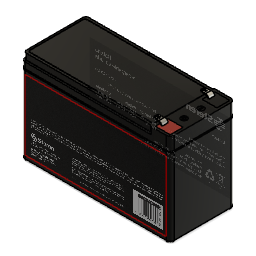
Batery-BR-1207-Steren v4 (Autodesk Fusion 360 design; units mm, degrees)
Autodesk Fusion 360 part; units mm, degrees
sketch "Sketch1" plane through (0, 0, 0) normal (0, 1, 0) x (1, 0, 0)
  line L0 (71, -32.5) -> (-71, -32.5)
  line L1 (-75, -28.5) -> (-75, 28.5)
  line L2 (-71, 32.5) -> (71, 32.5)
  line L3 (75, 28.5) -> (75, -28.5)
  line L4 (75, -32.5) -> (-75, 32.5) construction
  line L5 (-75, -32.5) -> (75, 32.5) construction
  arc A0 (-71, 32.5) -> (-75, 28.5) centre (-71, 28.5) ccw
  arc A1 (75, 28.5) -> (71, 32.5) centre (71, 28.5) ccw
  arc A2 (71, -32.5) -> (75, -28.5) centre (71, -28.5) ccw
  arc A3 (-75, -28.5) -> (-71, -32.5) centre (-71, -28.5) ccw
  dimension "d1" = 150
  dimension "d2" = 65
  dimension "d3" = 4
  constraint horizontal L0
  constraint perpendicular L0 L1
  constraint parallel L0 L2
  constraint parallel L1 L3
  constraint coincident L4 origin
  constraint coincident L5 origin
  constraint coincident L4.end L2
  constraint coincident L4.end L1
  constraint tangent L2 A0
  constraint tangent L1 A0
  constraint coincident L5.end L2
  constraint coincident L5.end L3
  constraint tangent L2 A1
  constraint tangent L3 A1
  constraint equal A0 A1
  constraint coincident L4.start L3
  constraint coincident L4.start L0
  constraint tangent L3 A2
  constraint tangent L0 A2
  constraint equal A0 A2
  constraint coincident L5.start L0
  constraint coincident L5.start L1
  constraint tangent L0 A3
  constraint tangent L1 A3
  constraint equal A0 A3
  measures "d1" distance of L4.end L5.end
  measures "d2" distance of L5.start L4.end
  measures "d3" radius of A0
extrude "Extrude1" add sketch "Sketch1" along normal blind 79 makes body 1
fillet "Fillet1" radius 2 8 edges at (75, 0, 0) (73.8284, 0, -31.3284) (0, 0, -32.5) (-73.8284, 0, -31.3284) (-75, 0, 0) (-73.8284, 0, 31.3284) (0, 0, 32.5) (73.8284, 0, 31.3284) on bodies 1
sketch "Sketch2" plane through (0, 0, 0) normal (0, -1, 0) x (1, 0, 0)
  line L0 (73, -28.5) -> (73, 28.5)
  arc A0 (73, 28.5) -> (71, 30.5) centre (71, 28.5) ccw
  line L1 (71, 30.5) -> (-71, 30.5)
  arc A1 (-71, 30.5) -> (-73, 28.5) centre (-71, 28.5) ccw
  line L2 (-73, 28.5) -> (-73, -28.5)
  arc A2 (-73, -28.5) -> (-71, -30.5) centre (-71, -28.5) ccw
  line L3 (-71, -30.5) -> (71, -30.5)
  arc A3 (71, -30.5) -> (73, -28.5) centre (71, -28.5) ccw
  line L4 (0, 0) -> (-72, 0) construction
  line L5 (-72, 0) -> (-72, 30) construction
  line L6 (-72, 30) -> (-63.5, 30)
  line L7 (-63.5, 30) -> (-63.5, 26.5)
  line L8 (-63.5, 26.5) -> (-72, 26.5)
  line L9 (-72, 26.5) -> (-72, 30)
  line L10 (-72, 30) -> (-72, 21.5)
  line L11 (-72, 21.5) -> (-68.5, 21.5)
  line L12 (-68.5, 21.5) -> (-68.5, 30)
  line L13 (-68.5, 30) -> (-72, 30)
  line L14 (-63.5, -30) -> (-63.5, -26.5)
  line L15 (-72, -26.5) -> (-72, -30)
  line L16 (-72, -30) -> (-63.5, -30)
  line L17 (-72, -21.5) -> (-68.5, -21.5)
  line L18 (-68.5, -21.5) -> (-68.5, -30)
  line L19 (-68.5, -30) -> (-72, -30)
  line L20 (-72, -30) -> (-72, -21.5)
  line L21 (-63.5, -26.5) -> (-72, -26.5)
  line L22 (0, 0) -> (0, 28.4251)
  line L23 (72, 21.5) -> (68.5, 21.5)
  line L24 (63.5, -30) -> (63.5, -26.5)
  line L25 (63.5, -26.5) -> (72, -26.5)
  line L26 (72, -21.5) -> (68.5, -21.5)
  line L27 (72, 26.5) -> (72, 30)
  line L28 (68.5, -21.5) -> (68.5, -30)
  line L29 (72, -26.5) -> (72, -30)
  line L30 (72, 30) -> (72, 21.5)
  line L31 (68.5, -30) -> (72, -30)
  line L32 (72, 30) -> (63.5, 30)
  line L33 (68.5, 21.5) -> (68.5, 30)
  line L34 (72, -30) -> (63.5, -30)
  line L35 (68.5, 30) -> (72, 30)
  line L36 (72, -30) -> (72, -21.5)
  line L37 (63.5, 26.5) -> (72, 26.5)
  line L38 (63.5, 30) -> (63.5, 26.5)
  point P0 (-71, -28.5)
  point P1 (71, -28.5)
  point P2 (71, -28.5)
  point P3 (71, 28.5)
  dimension "d8" = 72
  dimension "d9" = 30
  dimension "d10" = 8.5
  dimension "d11" = 3.5
  dimension "d12" = 8.5
  dimension "d13" = 3.5
  constraint coincident L4.start L22.start
  constraint horizontal L4
  constraint perpendicular L4 L5
  constraint perpendicular L6 L7
  constraint parallel L6 L8
  constraint parallel L7 L9
  constraint perpendicular L5 L6
  constraint perpendicular L10 L11
  constraint parallel L10 L12
  constraint parallel L11 L13
  constraint perpendicular L8 L10
  constraint symmetric A1.centre L4 P0
  constraint symmetric L4 L5.end L15.end
  constraint symmetric L4 L6.end L14.start
  constraint symmetric L4 L7.end L14.end
  constraint symmetric L4 L8.end L15.start
  constraint symmetric L4 L10.end L17.start
  constraint symmetric L4 L11.end L17.end
  constraint symmetric L4 L12.end L18.end
  constraint perpendicular L4 L22
  constraint symmetric A1.centre L22 P3
  constraint symmetric P0 L22 P2
  constraint symmetric L5.end L22 L27.end
  constraint symmetric L6.end L22 L32.end
  constraint symmetric L7.end L22 L37.start
  constraint symmetric L8.end L22 L27.start
  constraint symmetric L10.end L22 L23.start
  constraint symmetric L11.end L22 L23.end
  constraint symmetric L12.end L22 L33.end
  constraint symmetric L17.start L22 L26.start
  constraint symmetric L17.end L22 L26.end
  constraint symmetric L18.end L22 L28.end
  constraint symmetric L15.end L22 L29.end
  constraint symmetric L15.start L22 L25.end
  constraint symmetric L14.end L22 L24.end
  constraint symmetric L14.start L22 L24.start
  measures "d8" distance of L4.start L4.end
  measures "d9" distance of L4.end L5.end
  measures "d10" distance of L5.end L6.end
  measures "d11" distance of L5.end L8.end
  measures "d12" distance of L5.end L10.end
  measures "d13" distance of L10.end L11.end
extrude "Extrude2" add sketch "Sketch2" along normal blind 0.1 contours L6 L8 L9 L10 L12 L13 | L6 L7 L8 L12 | L8 L10 L11 L12 | L14 L16 L18 L21 | L15 L16 L18 L19 L20 L21 | L17 L18 L20 L21 | L23 L30 L33 L37 | L27 L30 L32 L33 L35 L37 | L32 L33 L37 L38 | L24 L25 L28 L34 | L25 L28 L29 L31 L34 L36 | L25 L26 L28 L36 bodies 1
sketch "Sketch3" plane through (0, 79, 0) normal (0, 1, 0) x (-1, 0, 0)
  arc A0 (71, -32.5) -> (75, -28.5) centre (71, -28.5) ccw
  line L0 (75, -28.5) -> (75, 28.5)
  arc A1 (75, 28.5) -> (71, 32.5) centre (71, 28.5) ccw
  line L1 (71, 32.5) -> (-71, 32.5)
  arc A2 (-71, 32.5) -> (-75, 28.5) centre (-71, 28.5) ccw
  line L2 (-75, 28.5) -> (-75, -28.5)
  arc A3 (-75, -28.5) -> (-71, -32.5) centre (-71, -28.5) ccw
  line L3 (-71, -32.5) -> (71, -32.5)
  arc A4 (74.5, 28.5) -> (71, 32) centre (71, 28.5) ccw
  line L4 (71, 32) -> (-71, 32)
  arc A5 (-71, 32) -> (-74.5, 28.5) centre (-71, 28.5) ccw
  line L5 (-74.5, 28.5) -> (-74.5, -28.5)
  arc A6 (-74.5, -28.5) -> (-71, -32) centre (-71, -28.5) ccw
  line L6 (-71, -32) -> (71, -32)
  arc A7 (71, -32) -> (74.5, -28.5) centre (71, -28.5) ccw
  line L7 (74.5, -28.5) -> (74.5, 28.5)
  dimension "d16" = -0.5
extrude "Extrude3" add sketch "Sketch3" along normal blind 1.5 contours A4 L4 A5 L5 A6 L6 A7 L7 bodies 1
sketch "Sketch6" plane through (0, 80.5, 0) normal (0, 1, 0) x (-1, 0, 0)
  line L0 (74.5, -28.5) -> (74.5, 28.5)
  arc A0 (74.5, 28.5) -> (71, 32) centre (71, 28.5) ccw
  line L1 (71, 32) -> (-71, 32)
  arc A1 (-71, 32) -> (-74.5, 28.5) centre (-71, 28.5) ccw
  line L2 (-74.5, 28.5) -> (-74.5, -28.5)
  arc A2 (-74.5, -28.5) -> (-71, -32) centre (-71, -28.5) ccw
  line L3 (-71, -32) -> (71, -32)
  arc A3 (71, -32) -> (74.5, -28.5) centre (71, -28.5) ccw
  line L4 (71, 32.5) -> (-71, 32.5)
  arc A4 (-71, 32.5) -> (-75, 28.5) centre (-71, 28.5) ccw
  line L5 (-75, 28.5) -> (-75, -28.5)
  arc A5 (-75, -28.5) -> (-71, -32.5) centre (-71, -28.5) ccw
  line L6 (-71, -32.5) -> (71, -32.5)
  arc A6 (71, -32.5) -> (75, -28.5) centre (71, -28.5) ccw
  line L7 (75, -28.5) -> (75, 28.5)
  arc A7 (75, 28.5) -> (71, 32.5) centre (71, 28.5) ccw
  dimension "d19" = 0.5
extrude "Extrude4" add sketch "Sketch6" along normal blind 7 contours L0 A0 L1 A1 L2 A2 L3 A3 | L4 A4 L5 A5 L6 A6 L7 A7 bodies 1
sketch "Sketch7" plane through (0, 87.5, 0) normal (0, 1, 0) x (-1, 0, 0)
  arc A0 (75, 28.5) -> (71, 32.5) centre (71, 28.5) ccw
  line L0 (71, 32.5) -> (-71, 32.5)
  arc A1 (-71, 32.5) -> (-75, 28.5) centre (-71, 28.5) ccw
  line L1 (-75, 28.5) -> (-75, -28.5)
  arc A2 (-75, -28.5) -> (-71, -32.5) centre (-71, -28.5) ccw
  line L2 (-71, -32.5) -> (71, -32.5)
  arc A3 (71, -32.5) -> (75, -28.5) centre (71, -28.5) ccw
  line L3 (75, -28.5) -> (75, 28.5)
  line L4 (73.75, -28.5) -> (73.75, 28.5)
  arc A4 (73.75, 28.5) -> (71, 31.25) centre (71, 28.5) ccw
  line L5 (71, 31.25) -> (-71, 31.25)
  arc A5 (-71, 31.25) -> (-73.75, 28.5) centre (-71, 28.5) ccw
  line L6 (-73.75, 28.5) -> (-73.75, -28.5)
  arc A6 (-73.75, -28.5) -> (-71, -31.25) centre (-71, -28.5) ccw
  line L7 (-71, -31.25) -> (71, -31.25)
  arc A7 (71, -31.25) -> (73.75, -28.5) centre (71, -28.5) ccw
  dimension "d22" = -1.25
extrude "Extrude5" add sketch "Sketch7" along normal blind 6 contours L4 A4 L5 A5 L6 A6 L7 A7 bodies 1
sketch "Sketch8" plane through (0, 87.5, 0) normal (0, 1, 0) x (-1, 0, 0)
  line L0 (71, -31.25) -> (-71, -31.25)
  arc A0 (-73.75, -28.5) -> (-71, -31.25) centre (-71, -28.5) ccw
  line L1 (-73.75, -28.5) -> (-73.75, 28.5)
  arc A1 (-71, 31.25) -> (-73.75, 28.5) centre (-71, 28.5) ccw
  line L2 (-71, 31.25) -> (71, 31.25)
  arc A2 (73.75, 28.5) -> (71, 31.25) centre (71, 28.5) ccw
  line L3 (73.75, 28.5) -> (73.75, -28.5)
  arc A3 (71, -31.25) -> (73.75, -28.5) centre (71, -28.5) ccw
  arc A4 (75, 28.5) -> (71, 32.5) centre (71, 28.5) ccw
  line L4 (71, 32.5) -> (-71, 32.5)
  arc A5 (-71, 32.5) -> (-75, 28.5) centre (-71, 28.5) ccw
  line L5 (-75, 28.5) -> (-75, -28.5)
  arc A6 (-75, -28.5) -> (-71, -32.5) centre (-71, -28.5) ccw
  line L6 (-71, -32.5) -> (71, -32.5)
  arc A7 (71, -32.5) -> (75, -28.5) centre (71, -28.5) ccw
  line L7 (75, -28.5) -> (75, 28.5)
  line L8 (-75, 0) -> (-54, 0)
  line L9 (-54, 0) -> (-54, -32.5)
  line L10 (-54, 0) -> (-54, 32.5)
  dimension "d25" = 21
  constraint midpoint L5 L8.start
  constraint perpendicular L5 L8
  constraint coincident L6 L9.end
  constraint perpendicular L6 L9
  constraint coincident L4 L10.end
  constraint perpendicular L4 L10
  measures "d25" distance of L8.start L8.end
extrude "Extrude6" add sketch "Sketch8" along normal blind 6 contours L0 A0 L1 L5 A6 L6 L8 L9 | L1 A1 L2 L4 A5 L5 L8 L10 bodies 1
sketch "Sketch9" plane through (0, 93.5, 0) normal (0, 1, 0) x (-1, 0, 0)
  arc A0 (71, -31.25) -> (73.75, -28.5) centre (71, -28.5) ccw
  line L0 (73.75, -28.5) -> (73.75, 28.5)
  arc A1 (73.75, 28.5) -> (71, 31.25) centre (71, 28.5) ccw
  line L1 (71, 31.25) -> (-54, 31.25)
  line L2 (-54, 31.25) -> (-54, 32.5)
  line L3 (-54, 32.5) -> (-71, 32.5)
  arc A2 (-71, 32.5) -> (-75, 28.5) centre (-71, 28.5) ccw
  line L4 (-75, 28.5) -> (-75, -28.5)
  arc A3 (-75, -28.5) -> (-71, -32.5) centre (-71, -28.5) ccw
  line L5 (-71, -32.5) -> (-54, -32.5)
  line L6 (-54, -32.5) -> (-54, -31.25)
  line L7 (-54, -31.25) -> (71, -31.25)
  line L8 (-75, -8.5) -> (-65, -8.5)
  line L9 (-65, -8.5) -> (-65, -32.5)
  circle A4 centre (-65, -8.5) radius 3
  line L10 (-75, 0) -> (-26.9263, 0) construction
  circle A5 centre (-65, 8.5) radius 3
  dimension "d29" = 10
  dimension "d30" = 24
  dimension "d31" = 6
  constraint coincident L4 L8.start
  constraint perpendicular L4 L8
  constraint perpendicular L8 L9
  constraint coincident L5 L9.end
  constraint coincident L8.end L9.start
  constraint midpoint L4 L10.start
  constraint perpendicular L4 L10
  constraint symmetric A4 L10 A5
  measures "d29" distance of L8.start L8.end
  measures "d30" distance of L8.end L9.end
  measures "d31" diameter of A4
extrude "Extrude7" cut sketch "Sketch9" against normal blind 0.3 contours L8 L9 A4 | L8 L9 A4 | A5 bodies 1
fillet "Fillet2" radius 1 5 edges at (-8.5, 87.5, -32.5) (-73.8284, 87.5, -31.3284) (-75, 87.5, 0) (-73.8284, 87.5, 31.3284) (-8.5, 87.5, 32.5) on bodies 1
fillet "Fillet3" radius 2 1 edges at (54, 90, 32.5) on bodies 1
fillet "Fillet3" radius 1 1 edges at (54, 90, -32.5) on bodies 1
sketch "Sketch10" plane through (0, 93.2, 0) normal (0, 1, 0) x (-1, 0, 0)
  circle A0 centre (-65, 8.5) radius 3
  line L0 (-64.5, 6.5) -> (-64.5, 10.5)
  arc A1 (-64.5, 10.5) -> (-65.5, 10.5) centre (-65, 10.5) ccw
  line L1 (-65.5, 10.5) -> (-65.5, 6.5)
  arc A2 (-65.5, 6.5) -> (-64.5, 6.5) centre (-65, 6.5) ccw
  line L2 (-65, 6.5) -> (-65, 10.5) construction
  line L3 (-63, 9) -> (-67, 9)
  arc A3 (-67, 9) -> (-67, 8) centre (-67, 8.5) ccw
  line L4 (-67, 8) -> (-63, 8)
  arc A4 (-63, 8) -> (-63, 9) centre (-63, 8.5) ccw
  line L5 (-63, 8.5) -> (-67, 8.5) construction
  point P0 (-65, 8.5)
  point P1 (-65, 8.5)
  dimension "d40" = 2
  dimension "d41" = 1
  constraint tangent L0 A1
  constraint tangent A1 L1
  constraint parallel L0 L1
  constraint tangent L1 A2
  constraint tangent L0 A2
  constraint vertical L2
  constraint coincident P0 A0.centre
  constraint midpoint L2 P1
  constraint tangent L3 A3
  constraint tangent A3 L4
  constraint parallel L3 L4
  constraint tangent L4 A4
  constraint tangent L3 A4
  constraint perpendicular L1 L5
  constraint coincident P1 P0
  constraint midpoint L5 P1
  measures "d40" distance of A1.centre P1
  measures "d41" diameter of A1
extrude "Extrude8" add sketch "Sketch10" along normal blind 0.3 contours L0 L1 A2 L4 | L0 L1 L3 L4 | L0 L3 L4 A4 | L0 A1 L1 L3 | L1 L3 A3 L4 bodies 1
sketch "Sketch11" plane through (0, 93.2, 0) normal (0, 1, 0) x (-1, 0, 0)
  circle A0 centre (-65, -8.5) radius 3
  line L0 (-64.5, -10.5) -> (-64.5, -6.5)
  arc A1 (-64.5, -6.5) -> (-65.5, -6.5) centre (-65, -6.5) ccw
  line L1 (-65.5, -6.5) -> (-65.5, -10.5)
  arc A2 (-65.5, -10.5) -> (-64.5, -10.5) centre (-65, -10.5) ccw
  line L2 (-65, -10.5) -> (-65, -6.5) construction
  point P0 (-65, -8.5)
  dimension "d44" = 2
  dimension "d45" = 1
  constraint tangent L0 A1
  constraint tangent A1 L1
  constraint parallel L0 L1
  constraint tangent L1 A2
  constraint tangent L0 A2
  constraint vertical L2
  constraint coincident P0 A0.centre
  constraint midpoint L2 P0
  measures "d44" distance of A1.centre P0
  measures "d45" diameter of A1
extrude "Extrude9" add sketch "Sketch11" along normal blind 0.3 contours L0 A1 L1 A2 bodies 1
sketch "Sketch12" plane through (0, 93.5, 0) normal (0, 1, 0) x (-1, 0, 0)
  circle A0 centre (-65, 8.5) radius 3
  circle A1 centre (-65, -8.5) radius 3
  arc A2 (-55, -32.5) -> (-54, -31.5) centre (-55, -31.5) ccw
  line L0 (-54, -31.5) -> (-54, -31.25)
  line L1 (-54, -31.25) -> (71, -31.25)
  arc A3 (71, -31.25) -> (73.75, -28.5) centre (71, -28.5) ccw
  line L2 (73.75, -28.5) -> (73.75, 28.5)
  arc A4 (73.75, 28.5) -> (71, 31.25) centre (71, 28.5) ccw
  line L3 (71, 31.25) -> (-54, 31.25)
  arc A5 (-54, 31.25) -> (-55.854, 32.5) centre (-55.854, 30.5) ccw
  line L4 (-55.854, 32.5) -> (-71, 32.5)
  arc A6 (-71, 32.5) -> (-75, 28.5) centre (-71, 28.5) ccw
  line L5 (-75, 28.5) -> (-75, -28.5)
  arc A7 (-75, -28.5) -> (-71, -32.5) centre (-71, -28.5) ccw
  line L6 (-71, -32.5) -> (-55, -32.5)
  line L7 (-75, 26.5) -> (-60, 26.5)
  line L8 (-60, 26.5) -> (-60, 32.5)
  line L9 (-60, 26.5) -> (-60.9, 26.5)
  line L10 (-60.9, 26.5) -> (-60.9, 20.5)
  line L11 (-60.9, 20.5) -> (-60, 20.5)
  line L12 (-60, 20.5) -> (-60, 26.5)
  line L13 (-75, 0) -> (-30, 0) construction
  line L14 (-60.9, -26.5) -> (-60.9, -20.5)
  line L15 (-60, -20.5) -> (-60, -26.5)
  line L16 (-60.9, -20.5) -> (-60, -20.5)
  line L17 (-60, -26.5) -> (-60.9, -26.5)
  dimension "d48" = 15
  dimension "d49" = 6
  dimension "d50" = 0.9
  dimension "d51" = 6
  constraint coincident L5 L7.start
  constraint perpendicular L5 L7
  constraint perpendicular L7 L8
  constraint coincident L4 L8.end
  constraint horizontal L9
  constraint vertical L10
  constraint horizontal L11
  constraint vertical L12
  constraint midpoint L5 L13.start
  constraint perpendicular L5 L13
  constraint symmetric L7.end L13 L15.end
  constraint symmetric L9.end L13 L14.start
  constraint symmetric L10.end L13 L14.end
  constraint symmetric L11.end L13 L15.start
  measures "d48" distance of L7.start L7.end
  measures "d49" distance of L7.end L8.end
  measures "d50" distance of L7.end L9.end
  measures "d51" distance of L7.end L11.end
extrude "Extrude10" add sketch "Sketch12" along normal blind 3 contours L7 L9 L10 L11 L12 | L14 L15 L16 L17 bodies 1
sketch "Sketch13" plane through (60, 0, 0) normal (-1, 0, 0) x (0, 0, 1)
  line L0 (-26.5, 93.5) -> (-20.5, 93.5)
  line L1 (-20.5, 93.5) -> (-20.5, 96.5)
  line L2 (-20.5, 96.5) -> (-26.5, 96.5)
  line L3 (-26.5, 96.5) -> (-26.5, 93.5)
  line L4 (-26.5, 96.5) -> (-20.5, 96.5)
  line L5 (-20.5, 96.5) -> (-20.5, 95.6)
  line L6 (-20.5, 95.6) -> (-26.5, 95.6)
  line L7 (-26.5, 95.6) -> (-26.5, 96.5)
  dimension "d54" = 6
  dimension "d55" = 0.9
  constraint horizontal L4
  constraint vertical L5
  constraint horizontal L6
  constraint vertical L7
  constraint coincident L2.end L3.start
  measures "d54" distance of L2.end L1.end
  measures "d55" distance of L2.end L6.end
extrude "Extrude11" add sketch "Sketch13" along normal blind 2.61 contours L1 L2 L3 L4 L5 L6 L7 bodies 1
sketch "Sketch14" plane through (60, 0, 0) normal (-1, 0, 0) x (0, 0, 1)
  line L0 (20.5, 93.5) -> (26.5, 93.5)
  line L1 (26.5, 93.5) -> (26.5, 96.5)
  line L2 (26.5, 96.5) -> (20.5, 96.5)
  line L3 (20.5, 96.5) -> (20.5, 93.5)
  line L4 (20.5, 96.5) -> (26.5, 96.5)
  line L5 (26.5, 96.5) -> (26.5, 95.6)
  line L6 (26.5, 95.6) -> (20.5, 95.6)
  line L7 (20.5, 95.6) -> (20.5, 96.5)
  dimension "d58" = 6
  dimension "d59" = 0.9
  constraint horizontal L4
  constraint vertical L5
  constraint horizontal L6
  constraint vertical L7
  constraint coincident L2.end L3.start
  measures "d58" distance of L2.end L1.end
  measures "d59" distance of L2.end L6.end
extrude "Extrude12" add sketch "Sketch14" along normal blind 2.61 contours L1 L2 L3 L4 L5 L6 L7 bodies 1
sketch "Sketch15" plane through (57.39, 0, 0) normal (-1, 0, 0) x (0, 0, 1)
  line L0 (-26.5, 95.6) -> (-20.5, 95.6)
  line L1 (-20.5, 95.6) -> (-20.5, 96.5)
  line L2 (-20.5, 96.5) -> (-26.5, 96.5)
  line L3 (-26.5, 96.5) -> (-26.5, 95.6)
  line L4 (-26.5, 96.5) -> (-20.5, 96.5)
  line L5 (-23.5, 96.5) -> (-23.5, 95.6)
  line L6 (-21, 95.6) -> (-26, 95.6)
  line L7 (-26, 95.6) -> (-26, 96.5)
  line L8 (-26, 96.5) -> (-21, 96.5)
  line L9 (-21, 96.5) -> (-21, 95.6)
  line L10 (-21, 95.6) -> (-26, 96.5) construction
  line L11 (-26, 95.6) -> (-21, 96.5) construction
  point P0 (-23.5, 96.05)
  dimension "d62" = 5
  dimension "d63" = 0.9
  constraint coincident L2.end L3.start
  constraint coincident L1.end L2.start
  constraint midpoint L2 L5.start
  constraint midpoint L0 L5.end
  constraint horizontal L6
  constraint perpendicular L6 L7
  constraint parallel L6 L8
  constraint parallel L7 L9
  constraint coincident L10 P0
  constraint coincident L11 P0
  constraint midpoint L5 P0
  measures "d62" distance of L7.end L8.end
  measures "d63" distance of L6.end L7.end
extrude "Extrude13" add sketch "Sketch15" along normal blind 6.3 contours L0 L2 L4 L5 L6 L7 L8 | L0 L2 L4 L5 L6 L8 L9 bodies 1
sketch "Sketch16" plane through (57.39, 0, 0) normal (-1, 0, 0) x (0, 0, 1)
  line L0 (20.5, 95.6) -> (26.5, 95.6)
  line L1 (26.5, 95.6) -> (26.5, 96.5)
  line L2 (26.5, 96.5) -> (20.5, 96.5)
  line L3 (20.5, 96.5) -> (20.5, 95.6)
  line L4 (20.5, 96.5) -> (26.5, 96.5)
  line L5 (23.5, 96.5) -> (23.5, 95.6)
  line L6 (26, 95.6) -> (21, 95.6)
  line L7 (21, 95.6) -> (21, 96.5)
  line L8 (21, 96.5) -> (26, 96.5)
  line L9 (26, 96.5) -> (26, 95.6)
  line L10 (26, 95.6) -> (21, 96.5) construction
  line L11 (21, 95.6) -> (26, 96.5) construction
  point P0 (23.5, 96.05)
  dimension "d66" = 5
  dimension "d67" = 0.9
  constraint coincident L2.end L3.start
  constraint coincident L1.end L2.start
  constraint midpoint L2 L5.start
  constraint midpoint L0 L5.end
  constraint horizontal L6
  constraint perpendicular L6 L7
  constraint parallel L6 L8
  constraint parallel L7 L9
  constraint coincident L10 P0
  constraint coincident L11 P0
  constraint midpoint L5 P0
  measures "d66" distance of L7.end L8.end
  measures "d67" distance of L6.end L7.end
extrude "Extrude14" add sketch "Sketch16" along normal blind 6.3 contours L0 L2 L4 L5 L6 L7 L8 | L0 L2 L4 L5 L6 L8 L9 bodies 1
sketch "Sketch17" plane through (0, 96.5, 0) normal (0, 1, 0) x (-1, 0, 0)
  line L0 (-57.39, -20.5) -> (-60.9, -20.5)
  line L1 (-60.9, -20.5) -> (-60.9, -26.5)
  line L2 (-60.9, -26.5) -> (-57.39, -26.5)
  line L3 (-57.39, -26.5) -> (-57.39, -26)
  line L4 (-57.39, -26) -> (-51.09, -26)
  line L5 (-51.09, -26) -> (-51.09, -21)
  line L6 (-51.09, -21) -> (-57.39, -21)
  line L7 (-57.39, -21) -> (-57.39, -20.5)
  line L8 (-57.39, -26) -> (-57.39, -21)
  line L9 (-57.39, -23.5) -> (-51.09, -23.5)
  line L10 (-55.49, -22.75) -> (-52.99, -22.75)
  line L11 (-52.99, -22.75) -> (-52.99, -24.25)
  line L12 (-52.99, -24.25) -> (-55.49, -24.25)
  line L13 (-55.49, -24.25) -> (-55.49, -22.75)
  line L14 (-55.49, -22.75) -> (-52.99, -24.25) construction
  line L15 (-52.99, -22.75) -> (-55.49, -24.25) construction
  point P0 (-54.24, -23.5)
  dimension "d70" = 2.5
  dimension "d71" = 1.5
  constraint coincident L3.end L4.start
  constraint coincident L6.end L7.start
  constraint midpoint L8 L9.start
  constraint midpoint L5 L9.end
  constraint horizontal L10
  constraint perpendicular L10 L11
  constraint parallel L10 L12
  constraint parallel L11 L13
  constraint coincident L14 P0
  constraint coincident L15 P0
  constraint midpoint L9 P0
  measures "d70" distance of L11.end L12.end
  measures "d71" distance of L10.end L11.end
extrude "Extrude15" cut sketch "Sketch17" against normal blind 2 contours L9 L10 L11 L13 | L9 L11 L12 L13 bodies 1
sketch "Sketch18" plane through (0, 96.5, 0) normal (0, 1, 0) x (-1, 0, 0)
  line L0 (-57.39, 26.5) -> (-60.9, 26.5)
  line L1 (-60.9, 26.5) -> (-60.9, 20.5)
  line L2 (-60.9, 20.5) -> (-57.39, 20.5)
  line L3 (-57.39, 20.5) -> (-57.39, 21)
  line L4 (-57.39, 21) -> (-51.09, 21)
  line L5 (-51.09, 21) -> (-51.09, 26)
  line L6 (-51.09, 26) -> (-57.39, 26)
  line L7 (-57.39, 26) -> (-57.39, 26.5)
  line L8 (-57.39, 21) -> (-57.39, 26)
  line L9 (-57.39, 23.5) -> (-51.09, 23.5)
  line L10 (-55.49, 24.25) -> (-52.99, 24.25)
  line L11 (-52.99, 24.25) -> (-52.99, 22.75)
  line L12 (-52.99, 22.75) -> (-55.49, 22.75)
  line L13 (-55.49, 22.75) -> (-55.49, 24.25)
  line L14 (-55.49, 24.25) -> (-52.99, 22.75) construction
  line L15 (-52.99, 24.25) -> (-55.49, 22.75) construction
  point P0 (-54.24, 23.5)
  dimension "d74" = 2.5
  dimension "d75" = 1.5
  constraint coincident L3.end L4.start
  constraint coincident L6.end L7.start
  constraint midpoint L8 L9.start
  constraint midpoint L5 L9.end
  constraint horizontal L10
  constraint perpendicular L10 L11
  constraint parallel L10 L12
  constraint parallel L11 L13
  constraint coincident L14 P0
  constraint coincident L15 P0
  constraint midpoint L9 P0
  measures "d74" distance of L11.end L12.end
  measures "d75" distance of L10.end L11.end
extrude "Extrude16" cut sketch "Sketch18" against normal blind 1.5 contours L9 L10 L11 L13 | L9 L11 L12 L13 bodies 1
chamfer "Chamfer1" distance 1 angle 45 2 edges at (51.09, 96.05, 26) (51.09, 96.05, 21) on bodies 1
chamfer "Chamfer2" distance 1 angle 45 2 edges at (51.09, 96.05, -26) (51.09, 96.05, -21) on bodies 1
chamfer "Chamfer3" distance 0.2 distance2 1.2 4 edges at (51.09, 96.5, -23.5) (51.09, 96.5, 23.5) (51.09, 95.6, -23.5) (51.09, 95.6, 23.5) measured on face at (51.09, 95.9, -23) measured on face at (51.09, 95.9, 24) measured on face at (51.09, 95.9, -23) measured on face at (51.09, 95.9, 24) on bodies 1
fillet "Fillet4" radius 3.5 4 edges at (60, 95.6, -23.5) (60.9, 96.5, -23.5) (60.9, 96.5, 23.5) (60, 95.6, 23.5) on bodies 1
sketch "Sketch19" plane through (0, 93.5, 0) normal (0, 1, 0) x (-1, 0, 0)
  line L0 (-60, -26.5) -> (-60.9, -26.5)
  line L1 (-60.9, -26.5) -> (-60.9, -20.5)
  line L2 (-60.9, -20.5) -> (-60, -20.5)
  line L3 (-60, -20.5) -> (-60, -26.5)
  line L4 (-60, 20.5) -> (-60.9, 20.5)
  line L5 (-60.9, 20.5) -> (-60.9, 26.5)
  line L6 (-60.9, 26.5) -> (-60, 26.5)
  line L7 (-60, 26.5) -> (-60, 20.5)
  circle A0 centre (-65, 8.5) radius 3
  circle A1 centre (-65, -8.5) radius 3
  arc A2 (-55, -32.5) -> (-54, -31.5) centre (-55, -31.5) ccw
  line L8 (-54, -31.5) -> (-54, -31.25)
  line L9 (-54, -31.25) -> (71, -31.25)
  arc A3 (71, -31.25) -> (73.75, -28.5) centre (71, -28.5) ccw
  line L10 (73.75, -28.5) -> (73.75, 28.5)
  arc A4 (73.75, 28.5) -> (71, 31.25) centre (71, 28.5) ccw
  line L11 (71, 31.25) -> (-54, 31.25)
  arc A5 (-54, 31.25) -> (-55.854, 32.5) centre (-55.854, 30.5) ccw
  line L12 (-55.854, 32.5) -> (-71, 32.5)
  arc A6 (-71, 32.5) -> (-75, 28.5) centre (-71, 28.5) ccw
  line L13 (-75, 28.5) -> (-75, -28.5)
  arc A7 (-75, -28.5) -> (-71, -32.5) centre (-71, -28.5) ccw
  line L14 (-71, -32.5) -> (-55, -32.5)
  line L15 (-75, -30) -> (-72.5, -30)
  line L16 (-72.5, -30) -> (-72.5, -32.5)
  line L17 (-72.5, -30) -> (-57.5, -30)
  line L18 (-57.5, -30) -> (-57.5, -17)
  line L19 (-57.5, -17) -> (-72.5, -17)
  line L20 (-72.5, -17) -> (-72.5, -30)
  line L21 (-65, -30) -> (-65, -17)
  line L22 (-72.5, -23.5) -> (-57.5, -23.5)
  line L23 (-75, 0) -> (-30, 0) construction
  line L24 (-72.5, 30) -> (-57.5, 30)
  line L25 (-57.5, 30) -> (-57.5, 17)
  line L26 (-57.5, 17) -> (-72.5, 17)
  line L27 (-72.5, 17) -> (-72.5, 30)
  dimension "d84" = 2.5
  dimension "d85" = 2.5
  dimension "d86" = 15
  dimension "d87" = 13
  constraint coincident L13 L15.start
  constraint perpendicular L13 L15
  constraint perpendicular L15 L16
  constraint coincident L14 L16.end
  constraint horizontal L17
  constraint vertical L18
  constraint horizontal L19
  constraint vertical L20
  constraint midpoint L17 L21.start
  constraint midpoint L19 L21.end
  constraint midpoint L20 L22.start
  constraint midpoint L18 L22.end
  constraint midpoint L13 L23.start
  constraint perpendicular L13 L23
  constraint symmetric L15.end L23 L24.start
  constraint symmetric L17.end L23 L24.end
  constraint symmetric L18.end L23 L25.end
  constraint symmetric L19.end L23 L26.end
  measures "d84" distance of L15.start L15.end
  measures "d85" distance of L15.end L16.end
  measures "d86" distance of L15.end L17.end
  measures "d87" distance of L15.end L19.end
extrude "Extrude17" cut sketch "Sketch19" against normal blind 0.01 contours L0 L1 L3 L17 L18 L21 L22 | L1 L2 L3 L18 L19 L21 L22 | L19 L20 L21 L22 | L17 L20 L21 L22 | L24 L25 L26 L27 bodies 1
sketch "Sketch20" plane through (0, 93.5, 0) normal (0, 1, 0) x (-1, 0, 0)
  line L0 (-57.5, 30) -> (-57.5, 17)
  line L1 (-57.5, 17) -> (-72.5, 17)
  line L2 (-72.5, 17) -> (-72.5, 30)
  line L3 (-72.5, 30) -> (-57.5, 30)
  line L4 (-57.5, -30) -> (-72.5, -30)
  line L5 (-72.5, -30) -> (-72.5, -17)
  line L6 (-72.5, -17) -> (-57.5, -17)
  line L7 (-57.5, -17) -> (-57.5, -30)
  circle A0 centre (-65, 8.5) radius 3
  circle A1 centre (-65, -8.5) radius 3
  arc A2 (-55, -32.5) -> (-54, -31.5) centre (-55, -31.5) ccw
  line L8 (-54, -31.5) -> (-54, -31.25)
  line L9 (-54, -31.25) -> (71, -31.25)
  arc A3 (71, -31.25) -> (73.75, -28.5) centre (71, -28.5) ccw
  line L10 (73.75, -28.5) -> (73.75, 28.5)
  arc A4 (73.75, 28.5) -> (71, 31.25) centre (71, 28.5) ccw
  line L11 (71, 31.25) -> (-54, 31.25)
  arc A5 (-54, 31.25) -> (-55.854, 32.5) centre (-55.854, 30.5) ccw
  line L12 (-55.854, 32.5) -> (-71, 32.5)
  arc A6 (-71, 32.5) -> (-75, 28.5) centre (-71, 28.5) ccw
  line L13 (-75, 28.5) -> (-75, -28.5)
  arc A7 (-75, -28.5) -> (-71, -32.5) centre (-71, -28.5) ccw
  line L14 (-71, -32.5) -> (-55, -32.5)
  line L15 (-52.25, 28.5) -> (69.75, 28.5)
  line L16 (71.75, 26.5) -> (71.75, -26.5)
  line L17 (69.75, -28.5) -> (-52.25, -28.5)
  line L18 (-54.25, -26.5) -> (-54.25, 26.5)
  line L19 (-54.25, 28.5) -> (71.75, -28.5) construction
  line L20 (71.75, 28.5) -> (-54.25, -28.5) construction
  line L21 (73.75, 0) -> (8.75, 0)
  arc A8 (69.75, -28.5) -> (71.75, -26.5) centre (69.75, -26.5) ccw
  arc A9 (-54.25, -26.5) -> (-52.25, -28.5) centre (-52.25, -26.5) ccw
  arc A10 (-52.25, 28.5) -> (-54.25, 26.5) centre (-52.25, 26.5) ccw
  arc A11 (71.75, 26.5) -> (69.75, 28.5) centre (69.75, 26.5) ccw
  line L22 (8.75, 0) -> (8.75, -28.5)
  line L23 (8.75, 0) -> (8.75, 28.5)
  arc A12 (72.05, 26.5) -> (69.75, 28.8) centre (69.75, 26.5) ccw
  line L24 (-52.25, 28.8) -> (69.75, 28.8)
  arc A13 (-52.25, 28.8) -> (-54.55, 26.5) centre (-52.25, 26.5) ccw
  line L25 (-54.55, -26.5) -> (-54.55, 26.5)
  arc A14 (-54.55, -26.5) -> (-52.25, -28.8) centre (-52.25, -26.5) ccw
  line L26 (69.75, -28.8) -> (-52.25, -28.8)
  arc A15 (69.75, -28.8) -> (72.05, -26.5) centre (69.75, -26.5) ccw
  line L27 (72.05, 26.5) -> (72.05, -26.5)
  line L28 (7.25, 29.5) -> (10.25, 29.5)
  line L29 (10.25, 29.5) -> (10.25, 27.5)
  line L30 (10.25, 27.5) -> (7.25, 27.5)
  line L31 (7.25, 27.5) -> (7.25, 29.5)
  line L32 (7.25, 29.5) -> (10.25, 27.5) construction
  line L33 (10.25, 29.5) -> (7.25, 27.5) construction
  line L34 (7.25, -27.5) -> (10.25, -27.5)
  line L35 (10.25, -27.5) -> (10.25, -29.5)
  line L36 (10.25, -29.5) -> (7.25, -29.5)
  line L37 (7.25, -29.5) -> (7.25, -27.5)
  line L38 (7.25, -27.5) -> (10.25, -29.5) construction
  line L39 (10.25, -27.5) -> (7.25, -29.5) construction
  point P0 (8.75, 0)
  point P1 (8.75, 28.5)
  point P2 (8.75, -28.5)
  dimension "d90" = 126
  dimension "d91" = 57
  dimension "d92" = 65
  dimension "d93" = 2
  dimension "d94" = -0.3
  dimension "d95" = 3
  dimension "d96" = 2
  dimension "d97" = 3
  dimension "d98" = 2
  constraint horizontal L15
  constraint perpendicular L15 L16
  constraint parallel L15 L17
  constraint parallel L16 L18
  constraint coincident L19 P0
  constraint coincident L20 P0
  constraint midpoint L10 L21.start
  constraint coincident P0 L21.end
  constraint perpendicular L16 L21
  constraint coincident L19.end L17
  constraint coincident L19.end L16
  constraint tangent L17 A8
  constraint tangent L16 A8
  constraint coincident L20.end L17
  constraint coincident L20.end L18
  constraint tangent L17 A9
  constraint tangent L18 A9
  constraint equal A8 A9
  constraint coincident L19.start L18
  constraint coincident L19.start L15
  constraint tangent L18 A10
  constraint tangent L15 A10
  constraint equal A8 A10
  constraint coincident L20.start L15
  constraint coincident L20.start L16
  constraint tangent L15 A11
  constraint tangent L16 A11
  constraint equal A8 A11
  constraint midpoint L17 P2
  constraint midpoint L15 P1
  constraint horizontal L28
  constraint perpendicular L28 L29
  constraint parallel L28 L30
  constraint parallel L29 L31
  constraint coincident L32 P1
  constraint coincident L33 P1
  constraint coincident P1 L23.end
  constraint horizontal L34
  constraint perpendicular L34 L35
  constraint parallel L34 L36
  constraint parallel L35 L37
  constraint coincident L38 P2
  constraint coincident L39 P2
  constraint coincident P2 L22.end
  measures "d90" distance of L19.end L20.end
  measures "d91" distance of L20.start L19.end
  measures "d92" distance of L21.start P0
  measures "d93" radius of A8
  measures "d95" distance of L29.end L30.end
  measures "d96" distance of L28.end L29.end
  measures "d97" distance of L35.end L36.end
  measures "d98" distance of L34.end L35.end
extrude "Extrude18" cut sketch "Sketch20" against normal blind 1 contours L15 L17 L18 A9 A10 L24 A13 L25 A14 L26 L31 L37 | L15 L24 L29 L31 | L24 L28 L29 L31 | L15 L16 L21 A11 A12 L24 L27 L29 | L17 L26 L35 L37 | L16 L17 L21 A8 L26 A15 L27 L35 | L26 L35 L36 L37 bodies 1
sketch "Sketch21" plane through (0, 0, 0) normal (0, -1, 0) x (1, 0, 0)
  line L0 (72, 30) -> (72, 21.5)
  line L1 (72, 21.5) -> (68.5, 21.5)
  line L2 (68.5, 21.5) -> (68.5, 26.5)
  line L3 (68.5, 26.5) -> (63.5, 26.5)
  line L4 (63.5, 26.5) -> (63.5, 30)
  line L5 (63.5, 30) -> (72, 30)
  line L6 (-63.5, 30) -> (-63.5, 26.5)
  line L7 (-63.5, 26.5) -> (-68.5, 26.5)
  line L8 (-68.5, 26.5) -> (-68.5, 21.5)
  line L9 (-68.5, 21.5) -> (-72, 21.5)
  line L10 (-72, 21.5) -> (-72, 30)
  line L11 (-72, 30) -> (-63.5, 30)
  line L12 (63.5, -30) -> (63.5, -26.5)
  line L13 (63.5, -26.5) -> (68.5, -26.5)
  line L14 (68.5, -26.5) -> (68.5, -21.5)
  line L15 (68.5, -21.5) -> (72, -21.5)
  line L16 (72, -21.5) -> (72, -30)
  line L17 (72, -30) -> (63.5, -30)
  line L18 (-72, -30) -> (-72, -21.5)
  line L19 (-72, -21.5) -> (-68.5, -21.5)
  line L20 (-68.5, -21.5) -> (-68.5, -26.5)
  line L21 (-68.5, -26.5) -> (-63.5, -26.5)
  line L22 (-63.5, -26.5) -> (-63.5, -30)
  line L23 (-63.5, -30) -> (-72, -30)
  line L24 (73, -28.5) -> (73, 28.5)
  arc A0 (73, 28.5) -> (71, 30.5) centre (71, 28.5) ccw
  line L25 (71, 30.5) -> (-71, 30.5)
  arc A1 (-71, 30.5) -> (-73, 28.5) centre (-71, 28.5) ccw
  line L26 (-73, 28.5) -> (-73, -28.5)
  arc A2 (-73, -28.5) -> (-71, -30.5) centre (-71, -28.5) ccw
  line L27 (-71, -30.5) -> (71, -30.5)
  arc A3 (71, -30.5) -> (73, -28.5) centre (71, -28.5) ccw
  line L28 (80, 230) -> (-70.876, 230)
  line L29 (-70.876, 230) -> (-70.876, 164.976)
  line L30 (-70.876, 164.976) -> (80, 164.976)
  line L31 (80, 164.976) -> (80, 230)
  dimension "d101" = 150.876
  dimension "d102" = 65.024
  constraint horizontal L28
  constraint vertical L29
  constraint horizontal L30
  constraint vertical L31
  measures "d101" distance of L28.start L28.end
  measures "d102" distance of L28.start L30.end
extrude "Extrude19" add sketch "Sketch21" against normal blind 100.076 separate body contours L28 L29 L30 L31 makes body 2
move_body "Move1" bodies 2 to x (1, 0, 0) y (0, 1, 0) z (0, 0, 1) at (-5, 0, -197.5)
hidden bodies 2
equation "d22 = ( -( 65 - 62.5 ) / 2 ) * 1 mm"
